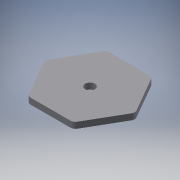
# Autodesk Inventor part: rotor 1
Saved by Autodesk Inventor 2017 (Build 210142000, 142)
## iProperties
Created: 2018-01-19
Part Number: rotor 1
Material: Generic
Document SubType Name: Modeling
Designer: RLanting
Density: 1 g/cm^3
Appearance: Default
Author: RLanting
Autodesk Inventor part; units mm, degrees
ref_plane "YZ Plane" through (0, 0, 0) normal (1, 0, 0) x (0, 1, 0)
ref_plane "XZ Plane" through (0, 0, 0) normal (0, 1, 0) x (-1, 0, 0)
ref_plane "XY Plane" through (0, 0, 0) normal (0, 0, 1) x (1, 0, 0)
sketch "Sketch1" plane through (0, 0, 0) normal (0, 0, 1) x (1, 0, 0)
  line L0 (-14.5, 25.1147) -> (14.5, 25.1147) construction
  line L1 (14.5, 25.1147) -> (29, 0) construction
  line L2 (29, 0) -> (14.5, -25.1147) construction
  line L3 (14.5, -25.1147) -> (-14.5, -25.1147) construction
  line L4 (-14.5, -25.1147) -> (-29, 0) construction
  line L5 (-29, 0) -> (-14.5, 25.1147) construction
  line L6 (-18.7639, 32.5) -> (18.7639, 32.5)
  line L7 (18.7639, 32.5) -> (37.5278, 0)
  line L8 (37.5278, 0) -> (18.7639, -32.5)
  line L9 (18.7639, -32.5) -> (-18.7639, -32.5)
  line L10 (-18.7639, -32.5) -> (-37.5278, 0)
  line L11 (-37.5278, 0) -> (-18.7639, 32.5)
  circle A0 centre (-14.5, 25.1147) radius 11 construction
  circle A1 centre (14.5, 25.1147) radius 11 construction
  circle A2 centre (29, 0) radius 11 construction
  circle A3 centre (14.5, -25.1147) radius 11 construction
  circle A4 centre (-14.5, -25.1147) radius 11 construction
  circle A5 centre (-29, 0) radius 11 construction
  circle A6 centre (-14.5, 25.1147) radius 1.35
  circle A7 centre (14.5, 25.1147) radius 1.35
  circle A8 centre (29, 0) radius 1.35
  circle A9 centre (14.5, -25.1147) radius 1.35
  circle A10 centre (-14.5, -25.1147) radius 1.35
  circle A11 centre (-29, 0) radius 1.35
  circle A12 centre (0, 0) radius 4
  circle A13 centre (0, 0) radius 40 construction
  dimension "d0" = 22
  dimension "d1" = 50.2295
  dimension "d2" = 2.7
  dimension "d3" = 65
  dimension "d4" = 8
  dimension "d8" = 80
  constraints: 24 end point, 16 coincident, 14 centre point, 10 equal radius, 2 horizontal, 1 tangent, 26 other
  measures "d0" diameter of A0
  measures "d1" distance between parallel lines of L3 L0
  measures "d2" diameter of A6
  measures "d3" distance between parallel lines of L9 L6
  measures "d4" diameter of A12
  measures "d8" diameter of A13
extrude "Extrusion1" add sketch "Sketch1" along normal blind 5
fillet "Fillet1" radius 4 6 edges at (37.5278, 0, 2.5) (18.7639, -32.5, 2.5) (-18.7639, -32.5, 2.5) (-37.5278, 0, 2.5) (-18.7639, 32.5, 2.5) (18.7639, 32.5, 2.5)
body "Solid1"
